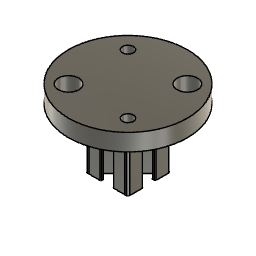
extrusion_peg (Autodesk Fusion 360 design; units mm, degrees)
Autodesk Fusion 360 part; units mm, degrees
note: some values were not read from the file. Chosen so that the rebuilt part matches the saved one: which bodies a step acts on.
sketch "Sketch1" plane through (0, 0, 0) normal (0, 0, 1) x (1, 0, 0)
  circle A0 centre (-17.5, -17.5) radius 3.25
  circle A1 centre (-17.5, 17.5) radius 6
  circle A2 centre (17.5, 17.5) radius 3.25
  circle A3 centre (17.5, -17.5) radius 6
  circle A4 centre (17.5, -17.5) radius 3.25
  circle A5 centre (-17.5, 17.5) radius 3.25
  circle A6 centre (0, 0) radius 35
  dimension "d2" = 360
  dimension "d3" = 70
  dimension "d4" = 17.5
  dimension "d5" = 17.5
  dimension "d6" = 6.5
  dimension "d7" = 12
  dimension "d8" = 12
  constraint coincident A6.centre origin
  constraint concentric A1 A5
  constraint concentric A3 A4
  measures "d3" diameter of A6
  measures "d4" vertical distance of A6.centre A2.centre
  measures "d5" horizontal distance of A6.centre A2.centre
  measures "d6" diameter of A2
  measures "d7" diameter of A1
  measures "d8" diameter of A3
extrude "Extrude1" add sketch "Sketch1" against normal blind 10 contours A6 makes body 1
sketch "Sketch2" plane through (0, 0, 0) normal (0, 0, 1) x (-1, 0, 0)
  circle A0 centre (17.5, 17.5) radius 3.25
  circle A1 centre (17.5, -17.5) radius 6
  circle A2 centre (-17.5, -17.5) radius 3.25
  circle A3 centre (-17.5, 17.5) radius 6
  circle A4 centre (0, 0) radius 35
  line L0 (-12.5, 12.5) -> (12.5, 12.5)
  line L1 (12.5, 12.5) -> (12.5, -12.5)
  line L2 (12.5, -12.5) -> (-12.5, -12.5)
  line L3 (-12.5, -12.5) -> (-12.5, 12.5)
  line L4 (-12.5, 12.5) -> (12.5, -12.5) construction
  line L5 (12.5, 12.5) -> (-12.5, -12.5) construction
  dimension "d11" = 25
  dimension "d12" = 25
  constraint horizontal L0
  constraint perpendicular L0 L1
  constraint parallel L0 L2
  constraint parallel L1 L3
  constraint coincident L4 A4.centre
  constraint coincident L5 A4.centre
  constraint coincident A4.centre origin
  measures "d11" distance of L0.end L1.end
  measures "d12" distance of L1 L3
extrude "Extrude2" add sketch "Sketch2" along normal blind 10 contours L0 L1 L2 L3 bodies 1
sketch "Sketch3" plane through (0, 0, 10) normal (0, 0, 1) x (-1, 0, 0)
  line L0 (-12.5, -12.5) -> (12.5, -12.5)
  line L1 (12.5, -12.5) -> (12.5, 12.5)
  line L2 (12.5, 12.5) -> (-12.5, 12.5)
  line L3 (-12.5, 12.5) -> (-12.5, -12.5)
  line L4 (-2.5858, -4) -> (2.5858, -4)
  line L5 (4, -2.5858) -> (4, 2.5858)
  line L6 (2.5858, 4) -> (-2.5858, 4)
  line L7 (-4, 2.5858) -> (-4, -2.5858)
  line L8 (-4, -4) -> (0, 0) construction
  line L9 (0, 0) -> (-4, 4) construction
  line L10 (12.5, -3.5) -> (12.5, -12.5)
  line L11 (3.5, -12.5) -> (3.5, -10.5)
  line L12 (3.5, -10.5) -> (9.0858, -10.5)
  line L13 (10.5, -9.0858) -> (10.5, -3.5)
  line L14 (10.5, -3.5) -> (12.5, -3.5)
  line L15 (10.5, -9.0858) -> (4, -2.5858)
  line L16 (9.0858, -10.5) -> (2.5858, -4)
  line L17 (12.5, -12.5) -> (3.5, -12.5)
  line L18 (9.0858, 10.5) -> (2.5858, 4)
  line L19 (10.5, 9.0858) -> (4, 2.5858)
  line L20 (10.5, 3.5) -> (10.5, 9.0858)
  line L21 (12.5, 3.5) -> (10.5, 3.5)
  line L22 (12.5, 12.5) -> (12.5, 3.5)
  line L23 (3.5, 12.5) -> (12.5, 12.5)
  line L24 (3.5, 10.5) -> (3.5, 12.5)
  line L25 (9.0858, 10.5) -> (3.5, 10.5)
  line L26 (-10.5, 9.0858) -> (-4, 2.5858)
  line L27 (-9.0858, 10.5) -> (-2.5858, 4)
  line L28 (-3.5, 10.5) -> (-9.0858, 10.5)
  line L29 (-3.5, 12.5) -> (-3.5, 10.5)
  line L30 (-12.5, 12.5) -> (-3.5, 12.5)
  line L31 (-12.5, 3.5) -> (-12.5, 12.5)
  line L32 (-10.5, 3.5) -> (-12.5, 3.5)
  line L33 (-10.5, 9.0858) -> (-10.5, 3.5)
  line L34 (-9.0858, -10.5) -> (-2.5858, -4)
  line L35 (-10.5, -9.0858) -> (-4, -2.5858)
  line L36 (-10.5, -3.5) -> (-10.5, -9.0858)
  line L37 (-12.5, -3.5) -> (-10.5, -3.5)
  line L38 (-12.5, -12.5) -> (-12.5, -3.5)
  line L39 (-3.5, -12.5) -> (-12.5, -12.5)
  line L40 (-3.5, -10.5) -> (-3.5, -12.5)
  line L41 (-9.0858, -10.5) -> (-3.5, -10.5)
  dimension "d16" = 8
  dimension "d17" = 2
  dimension "d18" = 2
  dimension "d19" = 2
  dimension "d20" = 9
  dimension "d21" = 9
  dimension "d22" = 135
  dimension "d24" = 360
  dimension "d25" = 8
  constraint horizontal L4
  constraint perpendicular L4 L5
  constraint parallel L4 L6
  constraint parallel L5 L7
  constraint coincident L8 L9.start
  constraint coincident L9 L8.end
  constraint coincident L8.end L9.start
  constraint coincident L1 L10.start
  constraint coincident L0.end L1.start
  constraint perpendicular L0 L10
  constraint coincident L0 L11.start
  constraint perpendicular L0 L11
  constraint perpendicular L11 L12
  constraint perpendicular L12 L13
  constraint perpendicular L1 L14
  constraint parallel L15 L16
  constraint symmetric L9 L15 L16
  measures "d16" distance of L8.start L9.end
  measures "d17" distance of L15 L16
  measures "d18" distance of L10.start L13.end
  measures "d19" distance of L11.start L11.end
  measures "d20" distance of L10 L11
  measures "d21" distance of L10.start L0.end
  measures "d22" angle of L5 L15
  measures "d25" distance of L5 L7
extrude "Extrude3" add sketch "Sketch3" along normal blind 50 contours L0 L1 L2 L3 L4 L5 L6 L7 L10 L11 L12 L13 L14 L15 L16 L17 L18 L19 L20 L21 L22 L23 L24 L25 L26 L27 L28 L29 L30 L31 L32 L33 L34 L35 L36 L37 L38 L39 L40 L41 bodies 1
fillet "Fillet1" radius 1 4 edges at (-12.5, -12.5, 30) (12.5, -12.5, 30) (12.5, 12.5, 30) (-12.5, 12.5, 30) on bodies 1
fillet "Fillet1" radius 0.5 24 edges at (-10.5, -3.5, 35) (-12.5, -3.5, 35) (-3.5, -10.5, 35) (-3.5, -12.5, 35) (-10.5, -9.0858, 35) (-9.0858, -10.5, 35) (10.5, -9.0858, 35) (9.0858, -10.5, 35) (10.5, -3.5, 35) (3.5, -10.5, 35) (3.5, -12.5, 35) (12.5, -3.5, 35) (10.5, 3.5, 35) (12.5, 3.5, 35) (10.5, 9.0858, 35) (9.0858, 10.5, 35) (3.5, 10.5, 35) (3.5, 12.5, 35) (-3.5, 12.5, 35) (-3.5, 10.5, 35) (-10.5, 3.5, 35) (-12.5, 3.5, 35) (-9.0858, 10.5, 35) (-10.5, 9.0858, 35) on bodies 1
fillet "Fillet1" radius 1 8 edges at (2.5858, -4, 35) (-2.5858, -4, 35) (4, -2.5858, 35) (4, 2.5858, 35) (2.5858, 4, 35) (-2.5858, 4, 35) (-4, -2.5858, 35) (-4, 2.5858, 35) on bodies 1
extrude "Extrude4" cut 1 faces at (1.3333, 0.7239, 60) along direction (0, 0, -1) blind 25 on bodies 1 bodies 1
split "Split1" by plane through (0, 0, 0) normal (0, 0, 1) bodies 1 makes body 2 at (12.5, 1.3333, 3.3333)
split "Split2" by plane through (0, 0, 10) normal (0, 0, 1) bodies 2 makes body 3 at (1.3333, 0.7239, 35)
split "Split3" by plane through (-10.5, 9.0858, 10) normal (1, 0, 0) and through (10.5, 3.5, 10) normal (-1, 0, 0) bodies 3 makes body 4 at (-12.5, 9, 26.6667) makes body 5 at (12.5, 9, 26.6667) makes body 6 at (12.5, -6.5, 18.3333) makes body 7 at (1.3333, 0.7239, 10)
split "Split4" by plane through (9.0858, 10.5, 10) normal (0, -1, 0) and through (-9.0858, -10.5, 10) normal (0, 1, 0) bodies 7 makes body 8 at (-6.1667, 12.5, 26.6667) makes body 9 at (6.1667, -12.5, 26.6667) makes body 10 at (-6.1667, -12.5, 18.3333) makes body 11 at (6.4477, -7.8619, 26.6667)
split "Split5" by plane through (-9.0858, -10.5, 10) normal (0.707107, -0.707107, 0) and through (-10.5, -9.0858, 10) normal (-0.707107, 0.707107, 0) bodies 11 makes body 12 at (10.5, 8.6834, 18.3333) makes body 13 at (6.4477, -7.8619, 26.6667) makes body 14 at (-8.6834, -10.5, 18.3333) makes body 15 at (8.281, 10.5, 18.3333) makes body 16 at (-6.4477, 7.8619, 18.3333) makes body 17 at (-10.5, -8.6834, 26.6667)
split "Split6" by plane through (-9.0858, 10.5, 10) normal (0.707107, 0.707107, 0) and through (-10.5, 9.0858, 10) normal (-0.707107, -0.707107, 0) bodies 16 makes body 18 at (0.7239, 4, 18.3333) makes body 19 at (-8.6834, 10.5, 18.3333) makes body 20 at (-4, 0.7239, 18.3333) makes body 21 at (-10.5, 8.281, 26.6667)
split "Split7" by plane through (10.5, -9.0858, 10) normal (0.707107, 0.707107, 0) and through (9.0858, -10.5, 10) normal (-0.707107, -0.707107, 0) bodies 13 makes body 22 at (4, -0.7239, 18.3333) makes body 23 at (10.5, -8.281, 26.6667) makes body 24 at (-0.7239, -4, 18.3333) makes body 25 at (8.281, -10.5, 18.3333)
split "Split8" by plane through (-2.5858, -4, 10) normal (0, -1, 0) bodies 24 makes body 26 at (2.781, -4.1953, 18.3333) makes body 27 at (-2.6333, -4.113, 18.3333)
split "Split9" by plane through (4, -2.5858, 10) normal (1, 0, 0) bodies 22 makes body 28 at (4.0237, -2.388, 18.3333) makes body 29 at (4.0463, 2.4723, 18.3333)
split "Split10" by plane through (2.5858, 4, 10) normal (0, 1, 0) bodies 18 makes body 30 at (-2.388, 4.0237, 18.3333) makes body 31 at (2.4723, 4.0463, 18.3333)
split "Split11" by plane through (-4, 2.5858, 10) normal (-1, 0, 0) bodies 20 makes body 32 at (-4.1953, 2.781, 26.6667) makes body 33 at (-4.0038, -2.2587, 18.3333)
move_body "Move1" bodies 2 29 18 27 16 24 6 15 5 12 3 25 22 31 17 4 8 9 10 21 28 26 30 19 32 20 23 11 33 13 1 7 14 to x (1, 0, 0) y (0, 1, 0) z (0, 0, 1) at (0, 0, -35)
move_body "Move2" bodies 23 3 17 27 30 28 12 2 9 10 25 13 24 33 14 4 5 18 6 20 22 32 21 19 15 26 8 29 16 1 7 11 31 to x (1, 0, 0) y (0, -1, 0) z (0, 0, -1) at (0, 0, 0)
move_body "Move3" bodies 14 25 2 26 24 32 10 13 33 28 1 3 30 16 8 27 22 23 21 20 29 11 9 17 4 15 19 5 6 7 31 18 12 to x (1, 0, 0) y (0, 1, 0) z (0, 0, 1) at (0, 0, -25)
named bodies: "Body2", "Body3", "Body4", "Body5", "Body6", "Body7", "Body8", "Body9", "Body10", "Body11", "Body12", "Body13", "Body14", "Body15", "Body16", "Body17", "Body18", "Body19", "Body20", "Body21", "Body22", "Body23", "Body24", "Body25", "Body26", "Body27", "Body28", "Body29", "Body30", "Body31", "Body32", "Body33"
